Autodesk Fusion 360 part; units mm, degrees
(part 4 of 8)
extrude "Extrude5" add sketch "Sketch4" along normal blind 3 separate body contours L966 L970 L974 L978 L982 L986 L990 L994 L998 L1002 L1006 L1010 L1014 L1018 L1022 L1026 L1030 L1034 L1038 L1042 L1046 L1050 L1054 L1058 L1062 L1066 L1076 L1077 L1078 L1079 L1080 L1081 L1082 L1083 L1084 L1085 L1086 L1087 L1088 L1089 L1090 L1091 L1092 L1093 L1094 L1095 L1096 L1097 L1098 L1099 L1100 L1101 L1102 L1103 L1104 L1105 L1106 L1107 L1108 L1109 L1110 L1111 L1112 L1113 L1114 L1115 L1116 L1117 L1118 L1119 L1120 L1121 L1122 L1123 L1124 L1125 L1126 L1127 L1128 L1129 L1130 L1131 L1132 L1133 L1134 L1135 L1136 L1137 L1138 L1139 L1140 L1141 L1142 L1143 L1144 L1145 L1146 L1147 L1148 L1149 L1150 L1151 L1152 L1153 L1154 L1155 L1156 L1157 L1158 L1159 L1160 L1161 L1162 L1163 L1164 L1165 L1166 L1167 L1168 L1169 L1170 L1171 L1172 L1173 L1174 L1175 L1176 L1177 L1178 L1179 L1180 L1181 L1182 L1183 L1184 L1185 L1186 L1187 L1188 L1189 L1190 L1191 L1192 L1193 L1194 L1195 L1196 L1197 L1198 L1199 L1200 L1201 L1202 L1203 L1204 L1205 L1206 L1207 L1208 L1209 L1210 L1211 L1212 L1213 L1214 L1215 L1216 L1217 L1218 L1219 L1220 L1221 L1222 L1223 L1224 L1225 L1226 L1227 L1228 L1229 L1230 L1231 L1232 L1233 L1234 L1235 L1236 L1237 L1238 L1239 L1240 L1241 L1242 L1243 L1244 L1245 L1246 L1247 L1248 L1249 L1250 L1251 L1252 L1253 L1254 L1255 L1256 L1257 L1258 L1259 L1260 L1261 L1262 L1263 L1264 L1265 L1266 L1267 L1268 L1269 L1270 L1271 L1272 L1273 L1274 L1275 L1276 L1277 L1278 L1279 L1280 L1281 L1282 L1283 L1284 L1285 L1286 L1287 L1288 L1289 L1290 L1291 L1292 L1293 L1294 L1295 L2115 L2119 makes body 5
extrude "Extrude6" add sketch "Sketch4" along normal blind 3 separate body contours L1289 L1293 L1503 L1507 L1511 L1515 L1519 L1523 L1527 L1531 L1535 L1539 L1543 L1547 L1551 L1555 L1559 L1563 L1567 L1571 L1575 L1579 L1583 L1587 L1591 L1595 L1599 L1908 L1909 L1910 L1911 L1912 L1913 L1914 L1915 L1916 L1917 L1918 L1919 L1920 L1921 L1922 L1923 L1924 L1925 L1926 L1927 L1928 L1929 L1930 L1931 L1932 L1933 L1934 L1935 L1936 L1937 L1938 L1939 L1940 L1941 L1942 L1943 L1944 L1945 L1946 L1947 L1948 L1949 L1950 L1951 L1952 L1953 L1954 L1955 L1956 L1957 L1958 L1959 L1960 L1961 L1962 L1963 L1964 L1965 L1966 L1967 L1968 L1969 L1970 L1971 L1972 L1973 L1974 L1975 L1976 L1977 L1978 L1979 L1980 L1981 L1982 L1983 L1984 L1985 L1986 L1987 L1988 L1989 L1990 L1991 L1992 L1993 L1994 L1995 L1996 L1997 L1998 L1999 L2000 L2001 L2002 L2003 L2004 L2005 L2006 L2007 L2008 L2009 L2010 L2011 L2012 L2013 L2014 L2015 L2016 L2017 L2018 L2019 L2020 L2021 L2022 L2023 L2024 L2025 L2026 L2027 L2028 L2029 L2030 L2031 L2032 L2033 L2034 L2035 L2036 L2037 L2038 L2039 L2040 L2041 L2042 L2043 L2044 L2045 L2046 L2047 L2048 L2049 L2050 L2051 L2052 L2053 L2054 L2055 L2056 L2057 L2058 L2059 L2060 L2061 L2062 L2063 L2064 L2065 L2066 L2067 L2068 L2069 L2070 L2071 L2072 L2073 L2074 L2075 L2076 L2077 L2078 L2079 L2080 L2081 L2082 L2083 L2084 L2085 L2086 L2087 L2088 L2089 L2090 L2091 L2092 L2093 L2094 L2095 L2096 L2097 L2098 L2099 L2100 L2101 L2102 L2103 L2104 L2105 L2106 L2107 L2108 L2109 L2110 L2111 L2112 L2113 L2114 L2115 L2116 L2117 L2118 L2119 L2120 L2121 L2122 L2123 L2124 L2125 L2126 L2127 L2128 L2129 L2130 L2131 L2132 L2133 L2134 L2135 L2136 L2137 L2138 L2139 L2140 L2141 L2142 L2143 L2144 L2145 L2146 L2147 L2148 L2149 L2150 L2151 L2152 L2153 L2154 L2155 L2156 L2157 L2158 L2159 L2160 L2161 L2162 L2163 L2164 L2165 L2166 L2167 L2168 L2169 L2170 L2171 L2172 L2173 L2174 L2175 L2176 L2177 L2178 L2179 L2180 L2181 L2182 L2183 L2184 L2185 L2186 L2187 L2188 L2189 L2190 L2191 L2192 L2193 L2194 L2195 L2196 L2197 L2198 L2199 L2200 L2201 L2202 L2203 L2204 L2205 L2206 L2207 L2208 L2209 L2210 L2211 L2212 L2213 L2214 L2215 L2216 L2217 L2218 L2219 L2220 L2221 L2222 L2223 L2224 L2225 L2226 L2227 L2228 L2229 L2230 L2231 L2232 L2233 L2234 L2235 L2236 L2237 L2238 L2239 L2240 L2241 L2242 L2243 L2244 L2245 L2246 L2247 L2248 L2249 L2250 L2251 L2252 L2253 L2254 L2255 L2256 L2257 L2258 L2259 L2260 L2261 L2262 L2263 L2264 L2265 L2266 L2267 L2268 L2269 L2270 L2271 L2272 L2273 L2274 L2275 L2276 L2277 L2278 L2279 L2280 L2281 L2282 L2283 L2284 L2285 L2286 L2287 L2288 L2289 L2290 L2291 L2292 L2293 L2294 L2295 L2296 L2297 L2298 L2299 L2300 L2301 L2302 L2303 L2304 L2305 L2306 L2307 L2308 L2309 L2310 L2311 L2312 L2313 L2314 L2315 L2316 L2317 L2318 L2319 L2320 L2321 L2322 L2323 L2324 L2325 L2326 L2327 L2328 L2329 L2330 L2331 L2332 L2333 L2334 L2335 L2336 L2337 L2338 L2339 L2340 L2341 L2342 L2343 L2344 L2345 L2346 L2347 L2348 L2349 L2350 L2351 L2352 L2353 L2354 L2355 L2356 L2357 L2358 L2359 L2360 L2361 L2362 L2363 L2364 L2365 L2366 L2367 L2368 L2369 L2370 L2371 L2372 L2373 L2374 L2375 L2376 L2377 L2378 L2379 L2380 L2381 L2382 L2383 L2384 L2385 L2386 L2387 L2388 L2389 L2390 L2391 L2392 L2393 L2394 L2395 L2396 L2397 L2398 L2399 L2400 L2401 L2402 L2403 L2404 L2405 L2406 L2407 L2408 L2409 L2410 L2411 L2412 L2413 L2414 L2415 L2416 L2417 L2418 L2419 L2420 L2421 L2422 L2423 L2424 L2425 L2426 L2427 L2428 L2429 L2430 L2431 L2432 L2433 L2434 L2435 L2436 L2437 L2438 L2439 L2440 L2441 L2442 L2443 L2444 L2445 L2446 L2447 L2448 L2449 L2450 L2451 L2452 L2453 L2454 L2455 L2456 L2457 L2458 L2459 L2460 L2461 L2462 L2463 L2464 L2465 L2466 L2467 L2468 L2469 L2470 L2471 L2472 L2473 L2474 L2475 L2476 L2477 L2478 L2479 L2480 L2481 L2482 L2483 L2484 L2485 L2486 L2487 L2488 L2489 L2490 L2491 L2492 L2493 L2494 L2495 L2496 L2497 L2498 L2499 L2500 L2501 L2502 L2503 L2504 L2505 L2506 L2507 L2508 L2509 L2510 L2511 L2512 L2513 L2514 L2515 L2516 L2517 L2518 L2519 makes body 6
extrude "Extrude7" cut sketch "Sketch5" along normal blind 90 bodies 1 6
sketch "Sketch6" plane through (0, 3, 0) normal (0, 1, 0) x (-1, 0, 0)
  line L0 (-641.3505, 34.85) -> (-638.3505, 34.85)
  line L1 (-638.3505, 34.85) -> (-638.3505, 38.6)
  line L2 (-638.3505, 38.6) -> (-641.3505, 38.6)
  line L3 (-641.3505, 38.6) -> (-641.3505, 42.35)
  line L4 (-641.3505, 42.35) -> (-642.1005, 42.35)
  line L5 (-642.1005, 42.35) -> (-642.1005, 39.35)
  line L6 (-642.1005, 39.35) -> (-645.8505, 39.35)
  line L7 (-645.8505, 39.35) -> (-645.8505, 42.35)
  line L8 (-645.8505, 42.35) -> (-648.8505, 42.35)
  line L9 (-648.8505, 42.35) -> (-648.8505, 39.35)
  line L10 (-648.8505, 39.35) -> (-651.8505, 39.35)
  line L11 (-651.8505, 39.35) -> (-651.8505, 42.35)
  line L12 (-651.8505, 42.35) -> (-654.8505, 42.35)
  line L13 (-654.8505, 42.35) -> (-654.8505, 39.35)
  line L14 (-654.8505, 39.35) -> (-657.8505, 39.35)
  line L15 (-657.8505, 39.35) -> (-657.8505, 42.35)
  line L16 (-657.8505, 42.35) -> (-660.8505, 42.35)
  line L17 (-660.8505, 42.35) -> (-660.8505, 39.35)
  line L18 (-660.8505, 39.35) -> (-663.8505, 39.35)
  line L19 (-663.8505, 39.35) -> (-663.8505, 42.35)
  line L20 (-663.8505, 42.35) -> (-666.8505, 42.35)
  line L21 (-666.8505, 42.35) -> (-666.8505, 39.35)
  line L22 (-666.8505, 39.35) -> (-669.8506, 39.35)
  line L23 (-669.8506, 39.35) -> (-669.8506, 42.35)
  line L24 (-669.8506, 42.35) -> (-672.8506, 42.35)
  line L25 (-672.8506, 42.35) -> (-672.8506, 39.35)
  line L26 (-672.8506, 39.35) -> (-675.8506, 39.35)
  line L27 (-675.8506, 39.35) -> (-675.8506, 42.35)
  line L28 (-675.8506, 42.35) -> (-678.8506, 42.35)
  line L29 (-678.8506, 42.35) -> (-678.8506, 39.35)
  line L30 (-678.8506, 39.35) -> (-681.8506, 39.35)
  line L31 (-681.8506, 39.35) -> (-681.8506, 42.35)
  line L32 (-681.8506, 42.35) -> (-684.8506, 42.35)
  line L33 (-684.8506, 42.35) -> (-684.8506, 39.35)
  line L34 (-684.8506, 39.35) -> (-687.8506, 39.35)
  line L35 (-687.8506, 39.35) -> (-687.8506, 42.35)
  line L36 (-687.8506, 42.35) -> (-690.8506, 42.35)
  line L37 (-690.8506, 42.35) -> (-690.8506, 39.35)
  line L38 (-690.8506, 39.35) -> (-693.8506, 39.35)
  line L39 (-693.8506, 39.35) -> (-693.8506, 42.35)
  line L40 (-693.8506, 42.35) -> (-696.8506, 42.35)
  line L41 (-696.8506, 42.35) -> (-696.8506, 39.35)
  line L42 (-696.8506, 39.35) -> (-699.8506, 39.35)
  line L43 (-699.8506, 39.35) -> (-699.8506, 42.35)
  line L44 (-699.8506, 42.35) -> (-702.8506, 42.35)
  line L45 (-702.8506, 42.35) -> (-702.8506, 39.35)
  line L46 (-702.8506, 39.35) -> (-705.8506, 39.35)
  line L47 (-705.8506, 39.35) -> (-705.8506, 42.35)
  line L48 (-705.8506, 42.35) -> (-708.8506, 42.35)
  line L49 (-708.8506, 42.35) -> (-708.8506, 39.35)
  line L50 (-708.8506, 39.35) -> (-711.8506, 39.35)
  line L51 (-711.8506, 39.35) -> (-711.8506, 42.35)
  line L52 (-711.8506, 42.35) -> (-714.8506, 42.35)
  line L53 (-714.8506, 42.35) -> (-714.8506, 39.35)
  line L54 (-714.8506, 39.35) -> (-717.8506, 39.35)
  line L55 (-717.8506, 39.35) -> (-717.8506, 42.35)
  line L56 (-717.8506, 42.35) -> (-720.8506, 42.35)
  line L57 (-720.8506, 42.35) -> (-720.8506, 39.35)
  line L58 (-720.8506, 39.35) -> (-723.8506, 39.35)
  line L59 (-723.8506, 39.35) -> (-723.8506, 42.35)
  line L60 (-723.8506, 42.35) -> (-726.8506, 42.35)
  line L61 (-726.8506, 42.35) -> (-726.8506, 39.35)
  line L62 (-726.8506, 39.35) -> (-729.8506, 39.35)
  line L63 (-729.8506, 39.35) -> (-729.8506, 42.35)
  line L64 (-729.8506, 42.35) -> (-732.8506, 42.35)
  line L65 (-732.8506, 42.35) -> (-732.8506, 39.35)
  line L66 (-732.8506, 39.35) -> (-735.8506, 39.35)
  line L67 (-735.8506, 39.35) -> (-735.8506, 42.35)
  line L68 (-735.8506, 42.35) -> (-738.8506, 42.35)
  line L69 (-738.8506, 42.35) -> (-738.8506, 39.35)
  line L70 (-738.8506, 39.35) -> (-741.8506, 39.35)
  line L71 (-741.8506, 39.35) -> (-741.8506, 42.35)
  line L72 (-741.8506, 42.35) -> (-744.8506, 42.35)
  line L73 (-744.8506, 42.35) -> (-744.8506, 39.35)
  line L74 (-744.8506, 39.35) -> (-747.8506, 39.35)
  line L75 (-747.8506, 39.35) -> (-747.8506, 42.35)
  line L76 (-747.8506, 42.35) -> (-750.8506, 42.35)
  line L77 (-750.8506, 42.35) -> (-750.8506, 39.35)
  line L78 (-750.8506, 39.35) -> (-753.8506, 39.35)
  line L79 (-753.8506, 39.35) -> (-753.8506, 42.35)
  line L80 (-753.8506, 42.35) -> (-756.8506, 42.35)
  line L81 (-756.8506, 42.35) -> (-756.8506, 39.35)
  line L82 (-756.8506, 39.35) -> (-759.8506, 39.35)
  line L83 (-759.8506, 39.35) -> (-759.8506, 42.35)
  line L84 (-759.8506, 42.35) -> (-762.8506, 42.35)
  line L85 (-762.8506, 42.35) -> (-762.8506, 39.35)
  line L86 (-762.8506, 39.35) -> (-765.8506, 39.35)
  line L87 (-765.8506, 39.35) -> (-765.8506, 42.35)
  line L88 (-765.8506, 42.35) -> (-768.8506, 42.35)
  line L89 (-768.8506, 42.35) -> (-768.8506, 39.35)
  line L90 (-768.8506, 39.35) -> (-771.8506, 39.35)
  line L91 (-771.8506, 39.35) -> (-771.8506, 42.35)
  line L92 (-771.8506, 42.35) -> (-774.8506, 42.35)
  line L93 (-774.8506, 42.35) -> (-774.8506, 39.35)
  line L94 (-774.8506, 39.35) -> (-777.8506, 39.35)
  line L95 (-777.8506, 39.35) -> (-777.8506, 42.35)
  line L96 (-777.8506, 42.35) -> (-780.8506, 42.35)
  line L97 (-780.8506, 42.35) -> (-780.8506, 39.35)
  line L98 (-780.8506, 39.35) -> (-783.8506, 39.35)
  line L99 (-783.8506, 39.35) -> (-783.8506, 42.35)
  line L100 (-783.8506, 42.35) -> (-786.8506, 42.35)
  line L101 (-786.8506, 42.35) -> (-786.8506, 39.35)
  line L102 (-786.8506, 39.35) -> (-790.6007, 39.35)
  line L103 (-790.6007, 39.35) -> (-790.6007, 42.35)
  line L104 (-790.6007, 42.35) -> (-791.3507, 42.35)
  line L105 (-791.3507, 42.35) -> (-791.3507, 38.6)
  line L106 (-791.3507, 38.6) -> (-794.3507, 38.6)
  line L107 (-794.3507, 38.6) -> (-794.3507, 34.85)
  line L108 (-794.3507, 34.85) -> (-791.3507, 34.85)
  line L109 (-791.3507, 34.85) -> (-791.3507, 31.85)
  line L110 (-791.3507, 31.85) -> (-794.3507, 31.85)
  line L111 (-794.3507, 31.85) -> (-794.3507, 28.1)
  line L112 (-794.3507, 28.1) -> (-791.3507, 28.1)
  line L113 (-791.3507, 28.1) -> (-791.3507, 24.35)
  line L114 (-791.3507, 24.35) -> (-790.6007, 24.35)
  line L115 (-790.6007, 24.35) -> (-790.6007, 27.35)
  line L116 (-790.6007, 27.35) -> (-786.8506, 27.35)
  line L117 (-786.8506, 27.35) -> (-786.8506, 24.35)
  line L118 (-786.8506, 24.35) -> (-783.8506, 24.35)
  line L119 (-783.8506, 24.35) -> (-783.8506, 27.35)
  line L120 (-783.8506, 27.35) -> (-780.8506, 27.35)
  line L121 (-780.8506, 27.35) -> (-780.8506, 24.35)
  line L122 (-780.8506, 24.35) -> (-777.8506, 24.35)
  line L123 (-777.8506, 24.35) -> (-777.8506, 27.35)
  line L124 (-777.8506, 27.35) -> (-774.8506, 27.35)
  line L125 (-774.8506, 27.35) -> (-774.8506, 24.35)
  line L126 (-774.8506, 24.35) -> (-771.8506, 24.35)
  line L127 (-771.8506, 24.35) -> (-771.8506, 27.35)
  line L128 (-771.8506, 27.35) -> (-768.8506, 27.35)
  line L129 (-768.8506, 27.35) -> (-768.8506, 24.35)
  line L130 (-768.8506, 24.35) -> (-765.8506, 24.35)
  line L131 (-765.8506, 24.35) -> (-765.8506, 27.35)
  line L132 (-765.8506, 27.35) -> (-762.8506, 27.35)
  line L133 (-762.8506, 27.35) -> (-762.8506, 24.35)
  line L134 (-762.8506, 24.35) -> (-759.8506, 24.35)
  line L135 (-759.8506, 24.35) -> (-759.8506, 27.35)
  line L136 (-759.8506, 27.35) -> (-756.8506, 27.35)
  line L137 (-756.8506, 27.35) -> (-756.8506, 24.35)
  line L138 (-756.8506, 24.35) -> (-753.8506, 24.35)
  line L139 (-753.8506, 24.35) -> (-753.8506, 27.35)
  line L140 (-753.8506, 27.35) -> (-750.8506, 27.35)
  line L141 (-750.8506, 27.35) -> (-750.8506, 24.35)
  line L142 (-750.8506, 24.35) -> (-747.8506, 24.35)
  line L143 (-747.8506, 24.35) -> (-747.8506, 27.35)
  line L144 (-747.8506, 27.35) -> (-744.8506, 27.35)
  line L145 (-744.8506, 27.35) -> (-744.8506, 24.35)
  line L146 (-744.8506, 24.35) -> (-741.8506, 24.35)
  line L147 (-741.8506, 24.35) -> (-741.8506, 27.35)
  line L148 (-741.8506, 27.35) -> (-738.8506, 27.35)
  line L149 (-738.8506, 27.35) -> (-738.8506, 24.35)
  line L150 (-738.8506, 24.35) -> (-735.8506, 24.35)
  line L151 (-735.8506, 24.35) -> (-735.8506, 27.35)
  line L152 (-735.8506, 27.35) -> (-732.8506, 27.35)
  line L153 (-732.8506, 27.35) -> (-732.8506, 24.35)
  line L154 (-732.8506, 24.35) -> (-729.8506, 24.35)
  line L155 (-729.8506, 24.35) -> (-729.8506, 27.35)
  line L156 (-729.8506, 27.35) -> (-726.8506, 27.35)
  line L157 (-726.8506, 27.35) -> (-726.8506, 24.35)
  line L158 (-726.8506, 24.35) -> (-723.8506, 24.35)
  line L159 (-723.8506, 24.35) -> (-723.8506, 27.35)
  line L160 (-723.8506, 27.35) -> (-720.8506, 27.35)
  line L161 (-720.8506, 27.35) -> (-720.8506, 24.35)
  line L162 (-720.8506, 24.35) -> (-717.8506, 24.35)
  line L163 (-717.8506, 24.35) -> (-717.8506, 27.35)
  line L164 (-717.8506, 27.35) -> (-714.8506, 27.35)
  line L165 (-714.8506, 27.35) -> (-714.8506, 24.35)
  line L166 (-714.8506, 24.35) -> (-711.8506, 24.35)
  line L167 (-711.8506, 24.35) -> (-711.8506, 27.35)
  line L168 (-711.8506, 27.35) -> (-708.8506, 27.35)
  line L169 (-708.8506, 27.35) -> (-708.8506, 24.35)
  line L170 (-708.8506, 24.35) -> (-705.8506, 24.35)
  line L171 (-705.8506, 24.35) -> (-705.8506, 27.35)
  line L172 (-705.8506, 27.35) -> (-702.8506, 27.35)
  line L173 (-702.8506, 27.35) -> (-702.8506, 24.35)
  line L174 (-702.8506, 24.35) -> (-699.8506, 24.35)
  line L175 (-699.8506, 24.35) -> (-699.8506, 27.35)
  line L176 (-699.8506, 27.35) -> (-696.8506, 27.35)
  line L177 (-696.8506, 27.35) -> (-696.8506, 24.35)
  line L178 (-696.8506, 24.35) -> (-693.8506, 24.35)
  line L179 (-693.8506, 24.35) -> (-693.8506, 27.35)
  line L180 (-693.8506, 27.35) -> (-690.8506, 27.35)
  line L181 (-690.8506, 27.35) -> (-690.8506, 24.35)
  line L182 (-690.8506, 24.35) -> (-687.8506, 24.35)
  line L183 (-687.8506, 24.35) -> (-687.8506, 27.35)
  line L184 (-687.8506, 27.35) -> (-684.8506, 27.35)
  line L185 (-684.8506, 27.35) -> (-684.8506, 24.35)
  line L186 (-684.8506, 24.35) -> (-681.8506, 24.35)
  line L187 (-681.8506, 24.35) -> (-681.8506, 27.35)
  line L188 (-681.8506, 27.35) -> (-678.8506, 27.35)
  line L189 (-678.8506, 27.35) -> (-678.8506, 24.35)
  line L190 (-678.8506, 24.35) -> (-675.8506, 24.35)
  line L191 (-675.8506, 24.35) -> (-675.8506, 27.35)
  line L192 (-675.8506, 27.35) -> (-672.8506, 27.35)
  line L193 (-672.8506, 27.35) -> (-672.8506, 24.35)
  line L194 (-672.8506, 24.35) -> (-669.8506, 24.35)
  line L195 (-669.8506, 24.35) -> (-669.8506, 27.35)
  line L196 (-669.8506, 27.35) -> (-666.8505, 27.35)
  line L197 (-666.8505, 27.35) -> (-666.8505, 24.35)
  line L198 (-666.8505, 24.35) -> (-663.8505, 24.35)
  line L199 (-663.8505, 24.35) -> (-663.8505, 27.35)
  line L200 (-663.8505, 27.35) -> (-660.8505, 27.35)
  line L201 (-660.8505, 27.35) -> (-660.8505, 24.35)
  line L202 (-660.8505, 24.35) -> (-657.8505, 24.35)
  line L203 (-657.8505, 24.35) -> (-657.8505, 27.35)
  line L204 (-657.8505, 27.35) -> (-654.8505, 27.35)
  line L205 (-654.8505, 27.35) -> (-654.8505, 24.35)
  line L206 (-654.8505, 24.35) -> (-651.8505, 24.35)
  line L207 (-651.8505, 24.35) -> (-651.8505, 27.35)
  line L208 (-651.8505, 27.35) -> (-648.8505, 27.35)
  line L209 (-648.8505, 27.35) -> (-648.8505, 24.35)
  line L210 (-648.8505, 24.35) -> (-645.8505, 24.35)
  line L211 (-645.8505, 24.35) -> (-645.8505, 27.35)
  line L212 (-645.8505, 27.35) -> (-642.1005, 27.35)
  line L213 (-642.1005, 27.35) -> (-642.1005, 24.35)
  line L214 (-642.1005, 24.35) -> (-641.3505, 24.35)
  line L215 (-641.3505, 24.35) -> (-641.3505, 28.1)
  line L216 (-641.3505, 28.1) -> (-638.3505, 28.1)
  line L217 (-638.3505, 28.1) -> (-638.3505, 31.85)
  line L218 (-638.3505, 31.85) -> (-641.3505, 31.85)
  line L219 (-641.3505, 31.85) -> (-641.3505, 34.85)
  line L220 (-712.1005, 38.1605) -> (-727.1005, 38.1605)
  line L221 (-727.1005, 38.1605) -> (-727.1005, 29.1605)
  line L222 (-727.1005, 29.1605) -> (-712.1005, 29.1605)
  line L223 (-712.1005, 29.1605) -> (-712.1005, 38.1605)
  dimension "d32" = 15
  dimension "d33" = 9
  dimension "d34" = 70
  measures "d32" distance of L220.start L220.end
  measures "d33" distance of L220.start L222.end
  measures "d34" distance of L5.end L220.start
extrude "Extrude8" cut sketch "Sketch6" against normal blind 30 contours L220 L221 L222 L223 bodies 5
sketch "Sketch7" plane through (0, 3, 0) normal (0, 1, 0) x (-1, 0, 0)
  line L0 (-319.3503, 31.85) -> (-322.3503, 31.85)
  line L1 (-322.3503, 31.85) -> (-322.3503, 28.1)
  line L2 (-322.3503, 28.1) -> (-319.3503, 28.1)
  line L3 (-319.3503, 28.1) -> (-319.3503, 27.35)
  line L4 (-319.3503, 27.35) -> (-317.6003, 27.35)
  line L5 (-317.6003, 27.35) -> (-317.6003, 24.35)
  line L6 (-317.6003, 24.35) -> (-312.8503, 24.35)
  line L7 (-312.8503, 24.35) -> (-312.8503, 27.35)
  line L8 (-312.8503, 27.35) -> (-309.8503, 27.35)
  line L9 (-309.8503, 27.35) -> (-309.8503, 24.35)
  line L10 (-309.8503, 24.35) -> (-306.8503, 24.35)
  line L11 (-306.8503, 24.35) -> (-306.8503, 27.35)
  line L12 (-306.8503, 27.35) -> (-303.8502, 27.35)
  line L13 (-303.8502, 27.35) -> (-303.8502, 24.35)
  line L14 (-303.8502, 24.35) -> (-300.8502, 24.35)
  line L15 (-300.8502, 24.35) -> (-300.8502, 27.35)
  line L16 (-300.8502, 27.35) -> (-297.8502, 27.35)
  line L17 (-297.8502, 27.35) -> (-297.8502, 24.35)
  line L18 (-297.8502, 24.35) -> (-294.8502, 24.35)
  line L19 (-294.8502, 24.35) -> (-294.8502, 27.35)
  line L20 (-294.8502, 27.35) -> (-291.8502, 27.35)
  line L21 (-291.8502, 27.35) -> (-291.8502, 24.35)
  line L22 (-291.8502, 24.35) -> (-288.8502, 24.35)
  line L23 (-288.8502, 24.35) -> (-288.8502, 27.35)
  line L24 (-288.8502, 27.35) -> (-285.8502, 27.35)
  line L25 (-285.8502, 27.35) -> (-285.8502, 24.35)
  line L26 (-285.8502, 24.35) -> (-282.8502, 24.35)
  line L27 (-282.8502, 24.35) -> (-282.8502, 27.35)
  line L28 (-282.8502, 27.35) -> (-279.8502, 27.35)
  line L29 (-279.8502, 27.35) -> (-279.8502, 24.35)
  line L30 (-279.8502, 24.35) -> (-276.8502, 24.35)
  line L31 (-276.8502, 24.35) -> (-276.8502, 27.35)
  line L32 (-276.8502, 27.35) -> (-273.8502, 27.35)
  line L33 (-273.8502, 27.35) -> (-273.8502, 24.35)
  line L34 (-273.8502, 24.35) -> (-270.8502, 24.35)
  line L35 (-270.8502, 24.35) -> (-270.8502, 27.35)
  line L36 (-270.8502, 27.35) -> (-267.8502, 27.35)
  line L37 (-267.8502, 27.35) -> (-267.8502, 24.35)
  line L38 (-267.8502, 24.35) -> (-264.8502, 24.35)
  line L39 (-264.8502, 24.35) -> (-264.8502, 27.35)
  line L40 (-264.8502, 27.35) -> (-261.8502, 27.35)
  line L41 (-261.8502, 27.35) -> (-261.8502, 24.35)
  line L42 (-261.8502, 24.35) -> (-258.8502, 24.35)
  line L43 (-258.8502, 24.35) -> (-258.8502, 27.35)
  line L44 (-258.8502, 27.35) -> (-255.8502, 27.35)
  line L45 (-255.8502, 27.35) -> (-255.8502, 24.35)
  line L46 (-255.8502, 24.35) -> (-252.8502, 24.35)
  line L47 (-252.8502, 24.35) -> (-252.8502, 27.35)
  line L48 (-252.8502, 27.35) -> (-249.8502, 27.35)
  line L49 (-249.8502, 27.35) -> (-249.8502, 24.35)
  line L50 (-249.8502, 24.35) -> (-246.8502, 24.35)
  line L51 (-246.8502, 24.35) -> (-246.8502, 27.35)
  line L52 (-246.8502, 27.35) -> (-243.8502, 27.35)
  line L53 (-243.8502, 27.35) -> (-243.8502, 24.35)
  line L54 (-243.8502, 24.35) -> (-240.8502, 24.35)
  line L55 (-240.8502, 24.35) -> (-240.8502, 27.35)
  line L56 (-240.8502, 27.35) -> (-237.8502, 27.35)
  line L57 (-237.8502, 27.35) -> (-237.8502, 24.35)
  line L58 (-237.8502, 24.35) -> (-234.8502, 24.35)
  line L59 (-234.8502, 24.35) -> (-234.8502, 27.35)
  line L60 (-234.8502, 27.35) -> (-231.8502, 27.35)
  line L61 (-231.8502, 27.35) -> (-231.8502, 24.35)
  line L62 (-231.8502, 24.35) -> (-228.8502, 24.35)
  line L63 (-228.8502, 24.35) -> (-228.8502, 27.35)
  line L64 (-228.8502, 27.35) -> (-225.8502, 27.35)
  line L65 (-225.8502, 27.35) -> (-225.8502, 24.35)
  line L66 (-225.8502, 24.35) -> (-222.8502, 24.35)
  line L67 (-222.8502, 24.35) -> (-222.8502, 27.35)
  line L68 (-222.8502, 27.35) -> (-219.8502, 27.35)
  line L69 (-219.8502, 27.35) -> (-219.8502, 24.35)
  line L70 (-219.8502, 24.35) -> (-216.8502, 24.35)
  line L71 (-216.8502, 24.35) -> (-216.8502, 27.35)
  line L72 (-216.8502, 27.35) -> (-213.8502, 27.35)
  line L73 (-213.8502, 27.35) -> (-213.8502, 24.35)
  line L74 (-213.8502, 24.35) -> (-210.8502, 24.35)
  line L75 (-210.8502, 24.35) -> (-210.8502, 27.35)
  line L76 (-210.8502, 27.35) -> (-207.8502, 27.35)
  line L77 (-207.8502, 27.35) -> (-207.8502, 24.35)
  line L78 (-207.8502, 24.35) -> (-204.8502, 24.35)
  line L79 (-204.8502, 24.35) -> (-204.8502, 27.35)
  line L80 (-204.8502, 27.35) -> (-201.8502, 27.35)
  line L81 (-201.8502, 27.35) -> (-201.8502, 24.35)
  line L82 (-201.8502, 24.35) -> (-198.8502, 24.35)
  line L83 (-198.8502, 24.35) -> (-198.8502, 27.35)
  line L84 (-198.8502, 27.35) -> (-195.8502, 27.35)
  line L85 (-195.8502, 27.35) -> (-195.8502, 24.35)
  line L86 (-195.8502, 24.35) -> (-192.8502, 24.35)
  line L87 (-192.8502, 24.35) -> (-192.8502, 27.35)
  line L88 (-192.8502, 27.35) -> (-189.8502, 27.35)
  line L89 (-189.8502, 27.35) -> (-189.8502, 24.35)
  line L90 (-189.8502, 24.35) -> (-186.8502, 24.35)
  line L91 (-186.8502, 24.35) -> (-186.8502, 27.35)
  line L92 (-186.8502, 27.35) -> (-183.8502, 27.35)
  line L93 (-183.8502, 27.35) -> (-183.8502, 24.35)
  line L94 (-183.8502, 24.35) -> (-180.8501, 24.35)
  line L95 (-180.8501, 24.35) -> (-180.8501, 27.35)
  line L96 (-180.8501, 27.35) -> (-177.8501, 27.35)
  line L97 (-177.8501, 27.35) -> (-177.8501, 24.35)
  line L98 (-177.8501, 24.35) -> (-174.8501, 24.35)
  line L99 (-174.8501, 24.35) -> (-174.8501, 27.35)
  line L100 (-174.8501, 27.35) -> (-171.8501, 27.35)
  line L101 (-171.8501, 27.35) -> (-171.8501, 24.35)
  line L102 (-171.8501, 24.35) -> (-168.8501, 24.35)
  line L103 (-168.8501, 24.35) -> (-168.8501, 27.35)
  line L104 (-168.8501, 27.35) -> (-165.8501, 27.35)
  line L105 (-165.8501, 27.35) -> (-165.8501, 24.35)
  line L106 (-165.8501, 24.35) -> (-162.8501, 24.35)
  line L107 (-162.8501, 24.35) -> (-162.8501, 27.35)
  line L108 (-162.8501, 27.35) -> (-159.8501, 27.35)
  line L109 (-159.8501, 27.35) -> (-159.8501, 24.35)
  line L110 (-159.8501, 24.35) -> (-156.8501, 24.35)
  line L111 (-156.8501, 24.35) -> (-156.8501, 27.35)
  line L112 (-156.8501, 27.35) -> (-153.8501, 27.35)
  line L113 (-153.8501, 27.35) -> (-153.8501, 24.35)
  line L114 (-153.8501, 24.35) -> (-150.8501, 24.35)
  line L115 (-150.8501, 24.35) -> (-150.8501, 27.35)
  line L116 (-150.8501, 27.35) -> (-147.8501, 27.35)
  line L117 (-147.8501, 27.35) -> (-147.8501, 24.35)
  line L118 (-147.8501, 24.35) -> (-144.8501, 24.35)
  line L119 (-144.8501, 24.35) -> (-144.8501, 27.35)
  line L120 (-144.8501, 27.35) -> (-141.8501, 27.35)
  line L121 (-141.8501, 27.35) -> (-141.8501, 24.35)
  line L122 (-141.8501, 24.35) -> (-138.8501, 24.35)
  line L123 (-138.8501, 24.35) -> (-138.8501, 27.35)
  line L124 (-138.8501, 27.35) -> (-135.8501, 27.35)
  line L125 (-135.8501, 27.35) -> (-135.8501, 24.35)
  line L126 (-135.8501, 24.35) -> (-132.8501, 24.35)
  line L127 (-132.8501, 24.35) -> (-132.8501, 27.35)
  line L128 (-132.8501, 27.35) -> (-129.8501, 27.35)
  line L129 (-129.8501, 27.35) -> (-129.8501, 24.35)
  line L130 (-129.8501, 24.35) -> (-126.8501, 24.35)
  line L131 (-126.8501, 24.35) -> (-126.8501, 27.35)
  line L132 (-126.8501, 27.35) -> (-123.8501, 27.35)
  line L133 (-123.8501, 27.35) -> (-123.8501, 24.35)
  line L134 (-123.8501, 24.35) -> (-120.8501, 24.35)
  line L135 (-120.8501, 24.35) -> (-120.8501, 27.35)
  line L136 (-120.8501, 27.35) -> (-117.8501, 27.35)
  line L137 (-117.8501, 27.35) -> (-117.8501, 24.35)
  line L138 (-117.8501, 24.35) -> (-114.8501, 24.35)
  line L139 (-114.8501, 24.35) -> (-114.8501, 27.35)
  line L140 (-114.8501, 27.35) -> (-111.8501, 27.35)
  line L141 (-111.8501, 27.35) -> (-111.8501, 24.35)
  line L142 (-111.8501, 24.35) -> (-108.8501, 24.35)
  line L143 (-108.8501, 24.35) -> (-108.8501, 27.35)
  line L144 (-108.8501, 27.35) -> (-105.8501, 27.35)
  line L145 (-105.8501, 27.35) -> (-105.8501, 24.35)
  line L146 (-105.8501, 24.35) -> (-102.8501, 24.35)
  line L147 (-102.8501, 24.35) -> (-102.8501, 27.35)
  line L148 (-102.8501, 27.35) -> (-99.8501, 27.35)
  line L149 (-99.8501, 27.35) -> (-99.8501, 24.35)
  line L150 (-99.8501, 24.35) -> (-96.8501, 24.35)
  line L151 (-96.8501, 24.35) -> (-96.8501, 27.35)
  line L152 (-96.8501, 27.35) -> (-93.8501, 27.35)
  line L153 (-93.8501, 27.35) -> (-93.8501, 24.35)
  line L154 (-93.8501, 24.35) -> (-90.8501, 24.35)
  line L155 (-90.8501, 24.35) -> (-90.8501, 27.35)
  line L156 (-90.8501, 27.35) -> (-87.8501, 27.35)
  line L157 (-87.8501, 27.35) -> (-87.8501, 24.35)
  line L158 (-87.8501, 24.35) -> (-84.8501, 24.35)
  line L159 (-84.8501, 24.35) -> (-84.8501, 27.35)
  line L160 (-84.8501, 27.35) -> (-81.8501, 27.35)
  line L161 (-81.8501, 27.35) -> (-81.8501, 24.35)
  line L162 (-81.8501, 24.35) -> (-78.8501, 24.35)
  line L163 (-78.8501, 24.35) -> (-78.8501, 27.35)
  line L164 (-78.8501, 27.35) -> (-75.8501, 27.35)
  line L165 (-75.8501, 27.35) -> (-75.8501, 24.35)
  line L166 (-75.8501, 24.35) -> (-72.8501, 24.35)
  line L167 (-72.8501, 24.35) -> (-72.8501, 27.35)
  line L168 (-72.8501, 27.35) -> (-69.8501, 27.35)
  line L169 (-69.8501, 27.35) -> (-69.8501, 24.35)
  line L170 (-69.8501, 24.35) -> (-66.8501, 24.35)
  line L171 (-66.8501, 24.35) -> (-66.8501, 27.35)
  line L172 (-66.8501, 27.35) -> (-63.8501, 27.35)
  line L173 (-63.8501, 27.35) -> (-63.8501, 24.35)
  line L174 (-63.8501, 24.35) -> (-60.8501, 24.35)
  line L175 (-60.8501, 24.35) -> (-60.8501, 27.35)
  line L176 (-60.8501, 27.35) -> (-57.85, 27.35)
  line L177 (-57.85, 27.35) -> (-57.85, 24.35)
  line L178 (-57.85, 24.35) -> (-54.85, 24.35)
  line L179 (-54.85, 24.35) -> (-54.85, 27.35)
  line L180 (-54.85, 27.35) -> (-51.85, 27.35)
  line L181 (-51.85, 27.35) -> (-51.85, 24.35)
  line L182 (-51.85, 24.35) -> (-48.85, 24.35)
  line L183 (-48.85, 24.35) -> (-48.85, 27.35)
  line L184 (-48.85, 27.35) -> (-45.85, 27.35)
  line L185 (-45.85, 27.35) -> (-45.85, 24.35)
  line L186 (-45.85, 24.35) -> (-42.85, 24.35)
  line L187 (-42.85, 24.35) -> (-42.85, 27.35)
  line L188 (-42.85, 27.35) -> (-39.85, 27.35)
  line L189 (-39.85, 27.35) -> (-39.85, 24.35)
  line L190 (-39.85, 24.35) -> (-36.85, 24.35)
  line L191 (-36.85, 24.35) -> (-36.85, 27.35)
  line L192 (-36.85, 27.35) -> (-33.85, 27.35)
  line L193 (-33.85, 27.35) -> (-33.85, 24.35)
  line L194 (-33.85, 24.35) -> (-30.85, 24.35)
  line L195 (-30.85, 24.35) -> (-30.85, 27.35)
  line L196 (-30.85, 27.35) -> (-27.85, 27.35)
  line L197 (-27.85, 27.35) -> (-27.85, 24.35)
  line L198 (-27.85, 24.35) -> (-24.85, 24.35)
  line L199 (-24.85, 24.35) -> (-24.85, 27.35)
  line L200 (-24.85, 27.35) -> (-21.85, 27.35)
  line L201 (-21.85, 27.35) -> (-21.85, 24.35)
  line L202 (-21.85, 24.35) -> (-18.85, 24.35)
  line L203 (-18.85, 24.35) -> (-18.85, 27.35)
  line L204 (-18.85, 27.35) -> (-15.85, 27.35)
  line L205 (-15.85, 27.35) -> (-15.85, 24.35)
  line L206 (-15.85, 24.35) -> (-11.1, 24.35)
  line L207 (-11.1, 24.35) -> (-11.1, 27.35)
  line L208 (-11.1, 27.35) -> (-9.35, 27.35)
  line L209 (-9.35, 27.35) -> (-9.35, 28.1)
  line L210 (-9.35, 28.1) -> (-6.35, 28.1)
  line L211 (-6.35, 28.1) -> (-6.35, 31.85)
  line L212 (-6.35, 31.85) -> (-9.35, 31.85)
  line L213 (-9.35, 31.85) -> (-9.35, 34.85)
  line L214 (-9.35, 34.85) -> (-6.35, 34.85)
  line L215 (-6.35, 34.85) -> (-6.35, 37.85)
  line L216 (-6.35, 37.85) -> (-9.35, 37.85)
  line L217 (-9.35, 37.85) -> (-9.35, 40.85)
  line L218 (-9.35, 40.85) -> (-6.35, 40.85)
  line L219 (-6.35, 40.85) -> (-6.35, 43.85)
  line L220 (-6.35, 43.85) -> (-9.35, 43.85)
  line L221 (-9.35, 43.85) -> (-9.35, 46.85)
  line L222 (-9.35, 46.85) -> (-6.35, 46.85)
  line L223 (-6.35, 46.85) -> (-6.35, 49.85)
  line L224 (-6.35, 49.85) -> (-9.35, 49.85)
  line L225 (-9.35, 49.85) -> (-9.35, 52.85)
  line L226 (-9.35, 52.85) -> (-6.35, 52.85)
  line L227 (-6.35, 52.85) -> (-6.35, 55.85)
  line L228 (-6.35, 55.85) -> (-9.35, 55.85)
  line L229 (-9.35, 55.85) -> (-9.35, 58.85)
  line L230 (-9.35, 58.85) -> (-6.35, 58.85)
  line L231 (-6.35, 58.85) -> (-6.35, 61.8501)
  line L232 (-6.35, 61.8501) -> (-9.35, 61.8501)
  line L233 (-9.35, 61.8501) -> (-9.35, 64.8501)
  line L234 (-9.35, 64.8501) -> (-6.35, 64.8501)
  line L235 (-6.35, 64.8501) -> (-6.35, 67.8501)
  line L236 (-6.35, 67.8501) -> (-9.35, 67.8501)
  line L237 (-9.35, 67.8501) -> (-9.35, 70.8501)
  line L238 (-9.35, 70.8501) -> (-6.35, 70.8501)
  line L239 (-6.35, 70.8501) -> (-6.35, 73.8501)
  line L240 (-6.35, 73.8501) -> (-9.35, 73.8501)
  line L241 (-9.35, 73.8501) -> (-9.35, 76.8501)
  line L242 (-9.35, 76.8501) -> (-6.35, 76.8501)
  line L243 (-6.35, 76.8501) -> (-6.35, 79.8501)
  line L244 (-6.35, 79.8501) -> (-9.35, 79.8501)
  line L245 (-9.35, 79.8501) -> (-9.35, 82.8501)
  line L246 (-9.35, 82.8501) -> (-6.35, 82.8501)
  line L247 (-6.35, 82.8501) -> (-6.35, 85.8501)
  line L248 (-6.35, 85.8501) -> (-9.35, 85.8501)
  line L249 (-9.35, 85.8501) -> (-9.35, 88.8501)
  line L250 (-9.35, 88.8501) -> (-6.35, 88.8501)
  line L251 (-6.35, 88.8501) -> (-6.35, 91.8501)
  line L252 (-6.35, 91.8501) -> (-9.35, 91.8501)
  line L253 (-9.35, 91.8501) -> (-9.35, 94.8501)
  line L254 (-9.35, 94.8501) -> (-6.35, 94.8501)
  line L255 (-6.35, 94.8501) -> (-6.35, 97.8501)
  line L256 (-6.35, 97.8501) -> (-9.35, 97.8501)
  line L257 (-9.35, 97.8501) -> (-9.35, 100.8501)
  line L258 (-9.35, 100.8501) -> (-6.35, 100.8501)
  line L259 (-6.35, 100.8501) -> (-6.35, 103.8501)
  line L260 (-6.35, 103.8501) -> (-9.35, 103.8501)
  line L261 (-9.35, 103.8501) -> (-9.35, 106.8501)
  line L262 (-9.35, 106.8501) -> (-6.35, 106.8501)
  line L263 (-6.35, 106.8501) -> (-6.35, 109.8501)
  line L264 (-6.35, 109.8501) -> (-9.35, 109.8501)
  line L265 (-9.35, 109.8501) -> (-9.35, 112.8501)
  line L266 (-9.35, 112.8501) -> (-6.35, 112.8501)
  line L267 (-6.35, 112.8501) -> (-6.35, 115.8501)
  line L268 (-6.35, 115.8501) -> (-9.35, 115.8501)
  line L269 (-9.35, 115.8501) -> (-9.35, 118.8501)
  line L270 (-9.35, 118.8501) -> (-6.35, 118.8501)
  line L271 (-6.35, 118.8501) -> (-6.35, 121.8501)
  line L272 (-6.35, 121.8501) -> (-9.35, 121.8501)
  line L273 (-9.35, 121.8501) -> (-9.35, 124.8501)
  line L274 (-9.35, 124.8501) -> (-6.35, 124.8501)
  line L275 (-6.35, 124.8501) -> (-6.35, 127.8501)
  line L276 (-6.35, 127.8501) -> (-9.35, 127.8501)
  line L277 (-9.35, 127.8501) -> (-9.35, 130.8501)
  line L278 (-9.35, 130.8501) -> (-6.35, 130.8501)
  line L279 (-6.35, 130.8501) -> (-6.35, 133.8501)
  line L280 (-6.35, 133.8501) -> (-9.35, 133.8501)
  line L281 (-9.35, 133.8501) -> (-9.35, 136.8501)
  line L282 (-9.35, 136.8501) -> (-6.35, 136.8501)
  line L283 (-6.35, 136.8501) -> (-6.35, 139.8501)
  line L284 (-6.35, 139.8501) -> (-9.35, 139.8501)
  line L285 (-9.35, 139.8501) -> (-9.35, 142.8501)
  line L286 (-9.35, 142.8501) -> (-6.35, 142.8501)
  line L287 (-6.35, 142.8501) -> (-6.35, 145.8501)
  line L288 (-6.35, 145.8501) -> (-9.35, 145.8501)
  line L289 (-9.35, 145.8501) -> (-9.35, 148.8501)
  line L290 (-9.35, 148.8501) -> (-6.35, 148.8501)
  line L291 (-6.35, 148.8501) -> (-6.35, 151.8501)
  line L292 (-6.35, 151.8501) -> (-9.35, 151.8501)
  line L293 (-9.35, 151.8501) -> (-9.35, 154.8501)
  line L294 (-9.35, 154.8501) -> (-6.35, 154.8501)
  line L295 (-6.35, 154.8501) -> (-6.35, 157.8501)
  line L296 (-6.35, 157.8501) -> (-9.35, 157.8501)
  line L297 (-9.35, 157.8501) -> (-9.35, 160.8501)
  line L298 (-9.35, 160.8501) -> (-6.35, 160.8501)
  line L299 (-6.35, 160.8501) -> (-6.35, 163.8501)
  line L300 (-6.35, 163.8501) -> (-9.35, 163.8501)
  line L301 (-9.35, 163.8501) -> (-9.35, 166.8501)
  line L302 (-9.35, 166.8501) -> (-6.35, 166.8501)
  line L303 (-6.35, 166.8501) -> (-6.35, 169.8501)
  line L304 (-6.35, 169.8501) -> (-9.35, 169.8501)
  line L305 (-9.35, 169.8501) -> (-9.35, 172.8501)
  line L306 (-9.35, 172.8501) -> (-6.35, 172.8501)
  line L307 (-6.35, 172.8501) -> (-6.35, 176.6001)
  line L308 (-6.35, 176.6001) -> (-9.35, 176.6001)
  line L309 (-9.35, 176.6001) -> (-9.35, 177.3501)
  line L310 (-9.35, 177.3501) -> (-11.1, 177.3501)
  line L311 (-11.1, 177.3501) -> (-11.1, 180.3501)
  line L312 (-11.1, 180.3501) -> (-15.85, 180.3501)
  line L313 (-15.85, 180.3501) -> (-15.85, 177.3501)
  line L314 (-15.85, 177.3501) -> (-18.85, 177.3501)
  line L315 (-18.85, 177.3501) -> (-18.85, 180.3501)
  line L316 (-18.85, 180.3501) -> (-21.85, 180.3501)
  line L317 (-21.85, 180.3501) -> (-21.85, 177.3501)
  line L318 (-21.85, 177.3501) -> (-24.85, 177.3501)
  line L319 (-24.85, 177.3501) -> (-24.85, 180.3501)
  line L320 (-24.85, 180.3501) -> (-27.85, 180.3501)
  line L321 (-27.85, 180.3501) -> (-27.85, 177.3501)
  line L322 (-27.85, 177.3501) -> (-30.85, 177.3501)
  line L323 (-30.85, 177.3501) -> (-30.85, 180.3501)
  line L324 (-30.85, 180.3501) -> (-33.85, 180.3501)
  line L325 (-33.85, 180.3501) -> (-33.85, 177.3501)
  line L326 (-33.85, 177.3501) -> (-36.85, 177.3501)
  line L327 (-36.85, 177.3501) -> (-36.85, 180.3501)
  line L328 (-36.85, 180.3501) -> (-39.85, 180.3501)
  line L329 (-39.85, 180.3501) -> (-39.85, 177.3501)
  line L330 (-39.85, 177.3501) -> (-42.85, 177.3501)
  line L331 (-42.85, 177.3501) -> (-42.85, 180.3501)
  line L332 (-42.85, 180.3501) -> (-45.85, 180.3501)
  line L333 (-45.85, 180.3501) -> (-45.85, 177.3501)
  line L334 (-45.85, 177.3501) -> (-48.85, 177.3501)
  line L335 (-48.85, 177.3501) -> (-48.85, 180.3501)
  line L336 (-48.85, 180.3501) -> (-51.85, 180.3501)
  line L337 (-51.85, 180.3501) -> (-51.85, 177.3501)
  line L338 (-51.85, 177.3501) -> (-54.85, 177.3501)
  line L339 (-54.85, 177.3501) -> (-54.85, 180.3501)
  line L340 (-54.85, 180.3501) -> (-57.85, 180.3501)
  line L341 (-57.85, 180.3501) -> (-57.85, 177.3501)
  line L342 (-57.85, 177.3501) -> (-60.8501, 177.3501)
  line L343 (-60.8501, 177.3501) -> (-60.8501, 180.3501)
  line L344 (-60.8501, 180.3501) -> (-63.8501, 180.3501)
  line L345 (-63.8501, 180.3501) -> (-63.8501, 177.3501)
  line L346 (-63.8501, 177.3501) -> (-66.8501, 177.3501)
  line L347 (-66.8501, 177.3501) -> (-66.8501, 180.3501)
  line L348 (-66.8501, 180.3501) -> (-69.8501, 180.3501)
  line L349 (-69.8501, 180.3501) -> (-69.8501, 177.3501)
  line L350 (-69.8501, 177.3501) -> (-72.8501, 177.3501)
  line L351 (-72.8501, 177.3501) -> (-72.8501, 180.3501)
  line L352 (-72.8501, 180.3501) -> (-75.8501, 180.3501)
  line L353 (-75.8501, 180.3501) -> (-75.8501, 177.3501)
  line L354 (-75.8501, 177.3501) -> (-78.8501, 177.3501)
  line L355 (-78.8501, 177.3501) -> (-78.8501, 180.3501)
  line L356 (-78.8501, 180.3501) -> (-81.8501, 180.3501)
  line L357 (-81.8501, 180.3501) -> (-81.8501, 177.3501)
  line L358 (-81.8501, 177.3501) -> (-84.8501, 177.3501)
  line L359 (-84.8501, 177.3501) -> (-84.8501, 180.3501)
  line L360 (-84.8501, 180.3501) -> (-87.8501, 180.3501)
  line L361 (-87.8501, 180.3501) -> (-87.8501, 177.3501)
  line L362 (-87.8501, 177.3501) -> (-90.8501, 177.3501)
  line L363 (-90.8501, 177.3501) -> (-90.8501, 180.3501)
  line L364 (-90.8501, 180.3501) -> (-93.8501, 180.3501)
  line L365 (-93.8501, 180.3501) -> (-93.8501, 177.3501)
  line L366 (-93.8501, 177.3501) -> (-96.8501, 177.3501)
  line L367 (-96.8501, 177.3501) -> (-96.8501, 180.3501)
  line L368 (-96.8501, 180.3501) -> (-99.8501, 180.3501)
  line L369 (-99.8501, 180.3501) -> (-99.8501, 177.3501)
  line L370 (-99.8501, 177.3501) -> (-102.8501, 177.3501)
  line L371 (-102.8501, 177.3501) -> (-102.8501, 180.3501)
  line L372 (-102.8501, 180.3501) -> (-105.8501, 180.3501)
  line L373 (-105.8501, 180.3501) -> (-105.8501, 177.3501)
  line L374 (-105.8501, 177.3501) -> (-108.8501, 177.3501)
  line L375 (-108.8501, 177.3501) -> (-108.8501, 180.3501)
  line L376 (-108.8501, 180.3501) -> (-111.8501, 180.3501)
  line L377 (-111.8501, 180.3501) -> (-111.8501, 177.3501)
  line L378 (-111.8501, 177.3501) -> (-114.8501, 177.3501)
  line L379 (-114.8501, 177.3501) -> (-114.8501, 180.3501)
  line L380 (-114.8501, 180.3501) -> (-117.8501, 180.3501)
  line L381 (-117.8501, 180.3501) -> (-117.8501, 177.3501)
  line L382 (-117.8501, 177.3501) -> (-120.8501, 177.3501)
  line L383 (-120.8501, 177.3501) -> (-120.8501, 180.3501)
  line L384 (-120.8501, 180.3501) -> (-123.8501, 180.3501)
  line L385 (-123.8501, 180.3501) -> (-123.8501, 177.3501)
  line L386 (-123.8501, 177.3501) -> (-126.8501, 177.3501)
  line L387 (-126.8501, 177.3501) -> (-126.8501, 180.3501)
  line L388 (-126.8501, 180.3501) -> (-129.8501, 180.3501)
  line L389 (-129.8501, 180.3501) -> (-129.8501, 177.3501)
  line L390 (-129.8501, 177.3501) -> (-132.8501, 177.3501)
  line L391 (-132.8501, 177.3501) -> (-132.8501, 180.3501)
  line L392 (-132.8501, 180.3501) -> (-135.8501, 180.3501)
  line L393 (-135.8501, 180.3501) -> (-135.8501, 177.3501)
  line L394 (-135.8501, 177.3501) -> (-138.8501, 177.3501)
  line L395 (-138.8501, 177.3501) -> (-138.8501, 180.3501)
  line L396 (-138.8501, 180.3501) -> (-141.8501, 180.3501)
  line L397 (-141.8501, 180.3501) -> (-141.8501, 177.3501)
  line L398 (-141.8501, 177.3501) -> (-144.8501, 177.3501)
  line L399 (-144.8501, 177.3501) -> (-144.8501, 180.3501)
  line L400 (-144.8501, 180.3501) -> (-147.8501, 180.3501)
  line L401 (-147.8501, 180.3501) -> (-147.8501, 177.3501)
  line L402 (-147.8501, 177.3501) -> (-150.8501, 177.3501)
  line L403 (-150.8501, 177.3501) -> (-150.8501, 180.3501)
  line L404 (-150.8501, 180.3501) -> (-153.8501, 180.3501)
  line L405 (-153.8501, 180.3501) -> (-153.8501, 177.3501)
  line L406 (-153.8501, 177.3501) -> (-156.8501, 177.3501)
  line L407 (-156.8501, 177.3501) -> (-156.8501, 180.3501)
  line L408 (-156.8501, 180.3501) -> (-159.8501, 180.3501)
  line L409 (-159.8501, 180.3501) -> (-159.8501, 177.3501)
  line L410 (-159.8501, 177.3501) -> (-162.8501, 177.3501)
  line L411 (-162.8501, 177.3501) -> (-162.8501, 180.3501)
  line L412 (-162.8501, 180.3501) -> (-165.8501, 180.3501)
  line L413 (-165.8501, 180.3501) -> (-165.8501, 177.3501)
  line L414 (-165.8501, 177.3501) -> (-168.8501, 177.3501)
  line L415 (-168.8501, 177.3501) -> (-168.8501, 180.3501)
  line L416 (-168.8501, 180.3501) -> (-171.8501, 180.3501)
  line L417 (-171.8501, 180.3501) -> (-171.8501, 177.3501)
  line L418 (-171.8501, 177.3501) -> (-174.8501, 177.3501)
  line L419 (-174.8501, 177.3501) -> (-174.8501, 180.3501)
  line L420 (-174.8501, 180.3501) -> (-177.8501, 180.3501)
  line L421 (-177.8501, 180.3501) -> (-177.8501, 177.3501)
  line L422 (-177.8501, 177.3501) -> (-180.8501, 177.3501)
  line L423 (-180.8501, 177.3501) -> (-180.8501, 180.3501)
  line L424 (-180.8501, 180.3501) -> (-183.8502, 180.3501)
  line L425 (-183.8502, 180.3501) -> (-183.8502, 177.3501)
  line L426 (-183.8502, 177.3501) -> (-186.8502, 177.3501)
  line L427 (-186.8502, 177.3501) -> (-186.8502, 180.3501)
  line L428 (-186.8502, 180.3501) -> (-189.8502, 180.3501)
  line L429 (-189.8502, 180.3501) -> (-189.8502, 177.3501)
  line L430 (-189.8502, 177.3501) -> (-192.8502, 177.3501)
  line L431 (-192.8502, 177.3501) -> (-192.8502, 180.3501)
  line L432 (-192.8502, 180.3501) -> (-195.8502, 180.3501)
  line L433 (-195.8502, 180.3501) -> (-195.8502, 177.3501)
  line L434 (-195.8502, 177.3501) -> (-198.8502, 177.3501)
  line L435 (-198.8502, 177.3501) -> (-198.8502, 180.3501)
  line L436 (-198.8502, 180.3501) -> (-201.8502, 180.3501)
  line L437 (-201.8502, 180.3501) -> (-201.8502, 177.3501)
  line L438 (-201.8502, 177.3501) -> (-204.8502, 177.3501)
  line L439 (-204.8502, 177.3501) -> (-204.8502, 180.3501)
  line L440 (-204.8502, 180.3501) -> (-207.8502, 180.3501)
  line L441 (-207.8502, 180.3501) -> (-207.8502, 177.3501)
  line L442 (-207.8502, 177.3501) -> (-210.8502, 177.3501)
  line L443 (-210.8502, 177.3501) -> (-210.8502, 180.3501)
  line L444 (-210.8502, 180.3501) -> (-213.8502, 180.3501)
  line L445 (-213.8502, 180.3501) -> (-213.8502, 177.3501)
  line L446 (-213.8502, 177.3501) -> (-216.8502, 177.3501)
  line L447 (-216.8502, 177.3501) -> (-216.8502, 180.3501)
  line L448 (-216.8502, 180.3501) -> (-219.8502, 180.3501)
  line L449 (-219.8502, 180.3501) -> (-219.8502, 177.3501)
  line L450 (-219.8502, 177.3501) -> (-222.8502, 177.3501)
  line L451 (-222.8502, 177.3501) -> (-222.8502, 180.3501)
  line L452 (-222.8502, 180.3501) -> (-225.8502, 180.3501)
  line L453 (-225.8502, 180.3501) -> (-225.8502, 177.3501)
  line L454 (-225.8502, 177.3501) -> (-228.8502, 177.3501)
  line L455 (-228.8502, 177.3501) -> (-228.8502, 180.3501)
  line L456 (-228.8502, 180.3501) -> (-231.8502, 180.3501)
  line L457 (-231.8502, 180.3501) -> (-231.8502, 177.3501)
  line L458 (-231.8502, 177.3501) -> (-234.8502, 177.3501)
  line L459 (-234.8502, 177.3501) -> (-234.8502, 180.3501)
  line L460 (-234.8502, 180.3501) -> (-237.8502, 180.3501)
  line L461 (-237.8502, 180.3501) -> (-237.8502, 177.3501)
  line L462 (-237.8502, 177.3501) -> (-240.8502, 177.3501)
  line L463 (-240.8502, 177.3501) -> (-240.8502, 180.3501)
  line L464 (-240.8502, 180.3501) -> (-243.8502, 180.3501)
  line L465 (-243.8502, 180.3501) -> (-243.8502, 177.3501)
  line L466 (-243.8502, 177.3501) -> (-246.8502, 177.3501)
  line L467 (-246.8502, 177.3501) -> (-246.8502, 180.3501)
  line L468 (-246.8502, 180.3501) -> (-249.8502, 180.3501)
  line L469 (-249.8502, 180.3501) -> (-249.8502, 177.3501)
  line L470 (-249.8502, 177.3501) -> (-252.8502, 177.3501)
  line L471 (-252.8502, 177.3501) -> (-252.8502, 180.3501)
  line L472 (-252.8502, 180.3501) -> (-255.8502, 180.3501)
  line L473 (-255.8502, 180.3501) -> (-255.8502, 177.3501)
  line L474 (-255.8502, 177.3501) -> (-258.8502, 177.3501)
  line L475 (-258.8502, 177.3501) -> (-258.8502, 180.3501)
  line L476 (-258.8502, 180.3501) -> (-261.8502, 180.3501)
  line L477 (-261.8502, 180.3501) -> (-261.8502, 177.3501)
  line L478 (-261.8502, 177.3501) -> (-264.8502, 177.3501)
  line L479 (-264.8502, 177.3501) -> (-264.8502, 180.3501)
  line L480 (-264.8502, 180.3501) -> (-267.8502, 180.3501)
  line L481 (-267.8502, 180.3501) -> (-267.8502, 177.3501)
  line L482 (-267.8502, 177.3501) -> (-270.8502, 177.3501)
  line L483 (-270.8502, 177.3501) -> (-270.8502, 180.3501)
  line L484 (-270.8502, 180.3501) -> (-273.8502, 180.3501)
  line L485 (-273.8502, 180.3501) -> (-273.8502, 177.3501)
  line L486 (-273.8502, 177.3501) -> (-276.8502, 177.3501)
  line L487 (-276.8502, 177.3501) -> (-276.8502, 180.3501)
  line L488 (-276.8502, 180.3501) -> (-279.8502, 180.3501)
  line L489 (-279.8502, 180.3501) -> (-279.8502, 177.3501)
  line L490 (-279.8502, 177.3501) -> (-282.8502, 177.3501)
  line L491 (-282.8502, 177.3501) -> (-282.8502, 180.3501)
  line L492 (-282.8502, 180.3501) -> (-285.8502, 180.3501)
  line L493 (-285.8502, 180.3501) -> (-285.8502, 177.3501)
  line L494 (-285.8502, 177.3501) -> (-288.8502, 177.3501)
  line L495 (-288.8502, 177.3501) -> (-288.8502, 180.3501)
  line L496 (-288.8502, 180.3501) -> (-291.8502, 180.3501)
  line L497 (-291.8502, 180.3501) -> (-291.8502, 177.3501)
  line L498 (-291.8502, 177.3501) -> (-294.8502, 177.3501)
  line L499 (-294.8502, 177.3501) -> (-294.8502, 180.3501)
  line L500 (-294.8502, 180.3501) -> (-297.8502, 180.3501)
  line L501 (-297.8502, 180.3501) -> (-297.8502, 177.3501)
  line L502 (-297.8502, 177.3501) -> (-300.8502, 177.3501)
  line L503 (-300.8502, 177.3501) -> (-300.8502, 180.3501)
  line L504 (-300.8502, 180.3501) -> (-303.8502, 180.3501)
  line L505 (-303.8502, 180.3501) -> (-303.8502, 177.3501)
  line L506 (-303.8502, 177.3501) -> (-306.8503, 177.3501)
  line L507 (-306.8503, 177.3501) -> (-306.8503, 180.3501)
  line L508 (-306.8503, 180.3501) -> (-309.8503, 180.3501)
  line L509 (-309.8503, 180.3501) -> (-309.8503, 177.3501)
  line L510 (-309.8503, 177.3501) -> (-312.8503, 177.3501)
  line L511 (-312.8503, 177.3501) -> (-312.8503, 180.3501)
  line L512 (-312.8503, 180.3501) -> (-317.6003, 180.3501)
  line L513 (-317.6003, 180.3501) -> (-317.6003, 177.3501)
  line L514 (-317.6003, 177.3501) -> (-319.3503, 177.3501)
  line L515 (-319.3503, 177.3501) -> (-319.3503, 176.6001)
  line L516 (-319.3503, 176.6001) -> (-322.3503, 176.6001)
  line L517 (-322.3503, 176.6001) -> (-322.3503, 172.8501)
  line L518 (-322.3503, 172.8501) -> (-319.3503, 172.8501)
  line L519 (-319.3503, 172.8501) -> (-319.3503, 169.8501)
  line L520 (-319.3503, 169.8501) -> (-322.3503, 169.8501)
  line L521 (-322.3503, 169.8501) -> (-322.3503, 166.8501)
  line L522 (-322.3503, 166.8501) -> (-319.3503, 166.8501)
  line L523 (-319.3503, 166.8501) -> (-319.3503, 163.8501)
  line L524 (-319.3503, 163.8501) -> (-322.3503, 163.8501)
  line L525 (-322.3503, 163.8501) -> (-322.3503, 160.8501)
  line L526 (-322.3503, 160.8501) -> (-319.3503, 160.8501)
  line L527 (-319.3503, 160.8501) -> (-319.3503, 157.8501)
  line L528 (-319.3503, 157.8501) -> (-322.3503, 157.8501)
  line L529 (-322.3503, 157.8501) -> (-322.3503, 154.8501)
  line L530 (-322.3503, 154.8501) -> (-319.3503, 154.8501)
  line L531 (-319.3503, 154.8501) -> (-319.3503, 151.8501)
  line L532 (-319.3503, 151.8501) -> (-322.3503, 151.8501)
  line L533 (-322.3503, 151.8501) -> (-322.3503, 148.8501)
  line L534 (-322.3503, 148.8501) -> (-319.3503, 148.8501)
  line L535 (-319.3503, 148.8501) -> (-319.3503, 145.8501)
  line L536 (-319.3503, 145.8501) -> (-322.3503, 145.8501)
  line L537 (-322.3503, 145.8501) -> (-322.3503, 142.8501)
  line L538 (-322.3503, 142.8501) -> (-319.3503, 142.8501)
  line L539 (-319.3503, 142.8501) -> (-319.3503, 139.8501)
  line L540 (-319.3503, 139.8501) -> (-322.3503, 139.8501)
  line L541 (-322.3503, 139.8501) -> (-322.3503, 136.8501)
  line L542 (-322.3503, 136.8501) -> (-319.3503, 136.8501)
  line L543 (-319.3503, 136.8501) -> (-319.3503, 133.8501)
  line L544 (-319.3503, 133.8501) -> (-322.3503, 133.8501)
  line L545 (-322.3503, 133.8501) -> (-322.3503, 130.8501)
  line L546 (-322.3503, 130.8501) -> (-319.3503, 130.8501)
  line L547 (-319.3503, 130.8501) -> (-319.3503, 127.8501)
  line L548 (-319.3503, 127.8501) -> (-322.3503, 127.8501)
  line L549 (-322.3503, 127.8501) -> (-322.3503, 124.8501)
  line L550 (-322.3503, 124.8501) -> (-319.3503, 124.8501)
  line L551 (-319.3503, 124.8501) -> (-319.3503, 121.8501)
  line L552 (-319.3503, 121.8501) -> (-322.3503, 121.8501)
  line L553 (-322.3503, 121.8501) -> (-322.3503, 118.8501)
  line L554 (-322.3503, 118.8501) -> (-319.3503, 118.8501)
  line L555 (-319.3503, 118.8501) -> (-319.3503, 115.8501)
  line L556 (-319.3503, 115.8501) -> (-322.3503, 115.8501)
  line L557 (-322.3503, 115.8501) -> (-322.3503, 112.8501)
  line L558 (-322.3503, 112.8501) -> (-319.3503, 112.8501)
  line L559 (-319.3503, 112.8501) -> (-319.3503, 109.8501)
  line L560 (-319.3503, 109.8501) -> (-322.3503, 109.8501)
  line L561 (-322.3503, 109.8501) -> (-322.3503, 106.8501)
  line L562 (-322.3503, 106.8501) -> (-319.3503, 106.8501)
  line L563 (-319.3503, 106.8501) -> (-319.3503, 103.8501)
  line L564 (-319.3503, 103.8501) -> (-322.3503, 103.8501)
  line L565 (-322.3503, 103.8501) -> (-322.3503, 100.8501)
  line L566 (-322.3503, 100.8501) -> (-319.3503, 100.8501)
  line L567 (-319.3503, 100.8501) -> (-319.3503, 97.8501)
  line L568 (-319.3503, 97.8501) -> (-322.3503, 97.8501)
  line L569 (-322.3503, 97.8501) -> (-322.3503, 94.8501)
  line L570 (-322.3503, 94.8501) -> (-319.3503, 94.8501)
  line L571 (-319.3503, 94.8501) -> (-319.3503, 91.8501)
  line L572 (-319.3503, 91.8501) -> (-322.3503, 91.8501)
  line L573 (-322.3503, 91.8501) -> (-322.3503, 88.8501)
  line L574 (-322.3503, 88.8501) -> (-319.3503, 88.8501)
  line L575 (-319.3503, 88.8501) -> (-319.3503, 85.8501)
  line L576 (-319.3503, 85.8501) -> (-322.3503, 85.8501)
  line L577 (-322.3503, 85.8501) -> (-322.3503, 82.8501)
  line L578 (-322.3503, 82.8501) -> (-319.3503, 82.8501)
  line L579 (-319.3503, 82.8501) -> (-319.3503, 79.8501)
  line L580 (-319.3503, 79.8501) -> (-322.3503, 79.8501)
  line L581 (-322.3503, 79.8501) -> (-322.3503, 76.8501)
  line L582 (-322.3503, 76.8501) -> (-319.3503, 76.8501)
  line L583 (-319.3503, 76.8501) -> (-319.3503, 73.8501)
  line L584 (-319.3503, 73.8501) -> (-322.3503, 73.8501)
  line L585 (-322.3503, 73.8501) -> (-322.3503, 70.8501)
  line L586 (-322.3503, 70.8501) -> (-319.3503, 70.8501)
  line L587 (-319.3503, 70.8501) -> (-319.3503, 67.8501)
  line L588 (-319.3503, 67.8501) -> (-322.3503, 67.8501)
  line L589 (-322.3503, 67.8501) -> (-322.3503, 64.8501)
  line L590 (-322.3503, 64.8501) -> (-319.3503, 64.8501)
  line L591 (-319.3503, 64.8501) -> (-319.3503, 61.8501)
  line L592 (-319.3503, 61.8501) -> (-322.3503, 61.8501)
  line L593 (-322.3503, 61.8501) -> (-322.3503, 58.85)